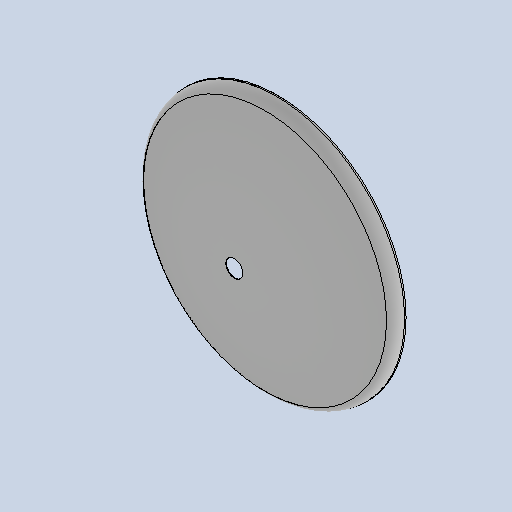
# Autodesk Inventor part: TKS 3901 dished head
Saved by Autodesk Inventor 2025.1 (Build 291241020, 241B)
## iProperties
Created: 2024-12-11
Part Number: TKS 3901 dished head
Material: Stainless Steel
Document SubType Name: Modeling
Designer: user
Density: 8 g/cm^3
Appearance: Default
Author: user
Autodesk Inventor part; units mm, degrees
ref_plane "YZ Plane" through (0, 0, 0) normal (1, 0, 0) x (0, 1, 0)
ref_plane "XZ Plane" through (0, 0, 0) normal (0, 1, 0) x (-1, 0, 0)
ref_plane "XY Plane" through (0, 0, 0) normal (0, 0, 1) x (1, 0, 0)
sketch "Sketch1" plane through (0, 0, 0) normal (0, 0, 1) x (1, 0, 0)
  line L0 (-1421.0526, 357.9157) -> (1421.0526, 357.9157) construction
  arc A0 (-1421.0526, 357.9157) -> (0, 0) centre (0, 3000) ccw construction
  line L1 (-1500, 490.0199) -> (1500, 490.0199) construction
  arc A1 (-1500, 490.0199) -> (-1421.0526, 357.9157) centre (-1350, 490.0199) ccw construction
  arc A2 (1421.0526, 357.9157) -> (1500, 490.0199) centre (1350, 490.0199) ccw
  line L2 (-1500, 490.0199) -> (-1500, 508.0199)
  line L3 (1500, 490.0199) -> (1500, 508.0199)
  line L4 (-1500, 508.0199) -> (0, 508.0199) construction
  line L5 (0, 508.0199) -> (0, 0)
  arc A3 (0, 0) -> (1421.0526, 357.9157) centre (0, 3000) ccw
  line L6 (0, 508.0199) -> (1500, 508.0199)
  dimension "d0" = 3000
  dimension "d1" = 150
  dimension "d2" = 18
  dimension "d3" = 3000
  dimension "d7_from_floor" = 0
  constraints: 14 end point, 8 point on circle, 4 centre point, 4 tangent, 3 horizontal, 3 vertical, 2 equal length, 1 equal radius, 1 point on line, 1 vertical alignment
  measures "d0" radius of A0
  measures "d1" radius of A1
  measures "d2" distance of L1.start L2.end
  measures "d3" distance of L1.start L1.end
  measures "d7_from_floor" distance of L5.end A0.end
revolve "Revolution1" add sketch "Sketch1" angle 360 about axis through (0, 508.0199, 0) along (0, -1, 0)
shell "Shell1" thickness 8 removed faces 1 at (349.4466, 508.0199, 349.2864)
sketch "Sketch2" plane through (0, 0, 0) normal (0, 1, 0) x (-1, 0, 0)
  circle A0 centre (0, 0) radius 100
  dimension "d10" = 200
  constraints: 1 centre point, 1 coincident
  measures "d10" diameter of A0
extrude "Extrusion1" cut sketch "Sketch2" along normal through all
equation "\"d0\" = d3"
equation "\"d3\" = MAIN_1_Filter_Diam"
equation "\"d10\" = MAIN_2_Outer_Tube_Diam"
equation "\"MAIN_1_Filter_Diam\" = 3000"
equation "\"MAIN_2_Outer_Tube_Diam\" = 200"
body "Solid1"
